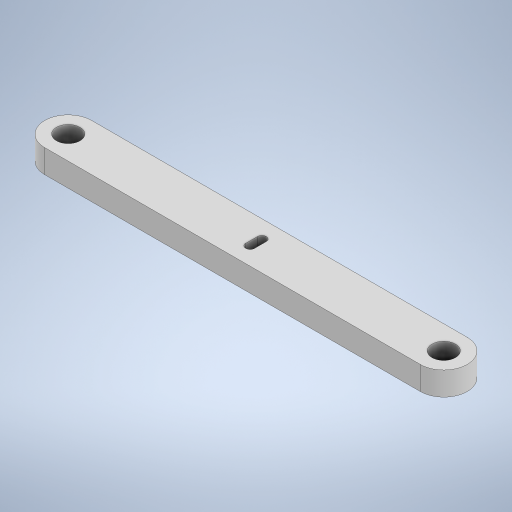
# Autodesk Inventor part: Langbektang houder
Saved by Autodesk Inventor 2023.2 (Build 272271000, 271)
## iProperties
Created: 2020-09-09
Part Number: Langbektang houder
Material: Generic
Document SubType Name: Modeling
Designer: nathan.bollaert
Density: 1 g/cm^3
Appearance: Default
Author: nathan.bollaert
Autodesk Inventor part; units mm, degrees
ref_plane "YZ Plane" through (0, 0, 0) normal (1, 0, 0) x (0, 1, 0)
ref_plane "XZ Plane" through (0, 0, 0) normal (0, 1, 0) x (-1, 0, 0)
ref_plane "XY Plane" through (0, 0, 0) normal (0, 0, 1) x (1, 0, 0)
sketch "Sketch1" plane through (0, 0, 0) normal (0, 1, 0) x (-1, 0, 0)
  circle A0 centre (-32, 0) radius 2
  circle A1 centre (32, 0) radius 2
  line L0 (32, 4) -> (-32, 4)
  line L1 (-32, -4) -> (32, -4)
  arc A2 (32, -4) -> (32, 4) centre (32, 0) ccw
  arc A3 (-32, 4) -> (-32, -4) centre (-32, 0) ccw
  line L2 (-0.75, -1) -> (-0.75, 1)
  line L3 (0.75, 1) -> (0.75, -1)
  line L4 (0.75, -1) -> (-0.75, 1) construction
  line L5 (-0.75, -1) -> (0.75, 1) construction
  arc A4 (0.75, 1) -> (-0.75, 1) centre (0, 1) ccw
  arc A5 (-0.75, -1) -> (0.75, -1) centre (0, -1) ccw
  point P0 (0, 0)
  dimension "d229" = 32
  dimension "d231" = 32
  dimension "d232" = 4
  dimension "d233" = 4
  dimension "d235" = 8
  dimension "d238" = 2
  dimension "d239" = 2
  dimension "d242" = 1.5
  dimension "d243" = 2
  constraints: 12 end point, 8 point on circle, 6 centre point, 4 tangent, 3 parallel, 2 horizontal alignment, 2 midpoint, 2 vertical alignment, 1 horizontal, 1 vertical
  measures "d229" distance of point (0, 0) A0.centre
  measures "d231" distance of A1.centre point (0, 0)
  measures "d232" diameter of A0
  measures "d233" diameter of A1
  measures "d235" distance of L1.start L0.end
  measures "d238" radial gap between concentric circles of A1 A2
  measures "d239" radial gap between concentric circles of A3 A0
  measures "d242" distance of L2.end L3.start
  measures "d243" distance of L2.start L2.end
extrude "Extrusion1" add sketch "Sketch1" along normal blind 4
body "Solid5"
